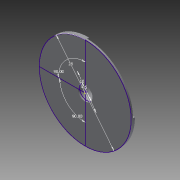
# Autodesk Inventor part: EncoderDisk
Saved by Autodesk Inventor 2014 SP1 (Build 180222100, 222)
## iProperties
Created: 2014-06-07
Part Number: EncoderDisk
Material: Generic
Document SubType Name: Modeling
Designer: Erin
Density: 1 g/cm^3
Appearance: Default
Author: Erin
Autodesk Inventor part; units mm, degrees
ref_plane "YZ Plane" through (0, 0, 0) normal (1, 0, 0) x (0, 1, 0)
ref_plane "XY Plane" through (0, 0, 0) normal (0, 0, 1) x (1, 0, 0)
sketch "Sketch1" plane through (0, 0, 0) normal (0, 1, 0) x (-1, 0, 0)
  arc A0 (0, 14) -> (0, -14) centre (0, 0) ccw
  line L0 (0, 0) -> (0, 14)
  line L1 (0, 0) -> (14, 0)
  arc A1 (14, 0) -> (0, 14) centre (0, 0) ccw
  line L2 (0, 0) -> (0, -14)
  arc A2 (0, -14) -> (14, 0) centre (0, 0) ccw
  dimension "d0" = 28
  dimension "d5" = 90
  dimension "d10" = 90
  constraints: 6 end point, 6 point on circle, 3 centre point, 1 coincident, 1 vertical
  measures "d0" diameter of A0
  measures "d5" angle of L1 L0
  measures "d10" angle of L2 L1
extrude "Extrusion1" add sketch "Sketch1" along normal blind 0.5
extrude "Extrusion2" add sketch "Sketch1" along normal blind 1.2 contours A1 L1 L0
extrude "Extrusion3" add sketch "Sketch1" along normal blind 0.6 contours L2 L1 A2
pattern_circular "Circular Pattern1" count 2 over 360 about axis through (0, -10, 0) along (0, 1, 0) of "Extrusion2", "Extrusion3"
ref_plane "Work Plane1" through (0, 0.5, 0) normal (0, 1, 0) x (-1, 0, 0)
sketch "Sketch2" plane through (0, 0.5, 0) normal (0, 1, 0) x (-1, 0, 0)
  circle A0 centre (0, 0) radius 5
  circle A1 centre (0, 0) radius 2.25
  dimension "d17" = 10
  dimension "d20" = 4.5
  constraints: 2 centre point, 2 coincident
  measures "d17" diameter of A0
  measures "d20" diameter of A1
extrude "Extrusion4" cut sketch "Sketch2" along normal blind 2 contours A0 | A1
extrude "Extrusion5" cut sketch "Sketch2" along normal mid plane 5 contours A1
extrude "Extrusion6" add sketch "Sketch2" along normal blind 2.5
body "Solid1"
